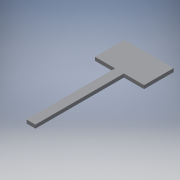
# Autodesk Inventor part: Bevestiging Token
Saved by Autodesk Inventor 2018.3 (Build 223284000, 284)
## iProperties
Created: 2020-12-14
Part Number: Bevestiging Token
Material: Generic
Document SubType Name: Modeling
Designer: daanv
Density: 1 g/cm^3
Appearance: Default
Author: daanv
Autodesk Inventor part; units mm, degrees
ref_plane "YZ Plane" through (0, 0, 0) normal (1, 0, 0) x (0, 1, 0)
ref_plane "XZ Plane" through (0, 0, 0) normal (0, 1, 0) x (-1, 0, 0)
ref_plane "XY Plane" through (0, 0, 0) normal (0, 0, 1) x (1, 0, 0)
sketch "Sketch1" plane through (0, 0, 0) normal (0, 0, 1) x (1, 0, 0)
  line L0 (0, 0) -> (1.8, 0)
  line L1 (1.8, 0) -> (1.8, 18)
  line L2 (1.8, 18) -> (0, 18)
  line L3 (0, 18) -> (0, 0)
  line L4 (-4.1, 18) -> (5.9, 18)
  line L5 (5.9, 18) -> (5.9, 24)
  line L6 (5.9, 24) -> (-4.1, 24)
  line L7 (-4.1, 24) -> (-4.1, 18)
  dimension "d0" = 1.8
  dimension "d1" = 18
  dimension "d2" = 10
  dimension "d3" = 6
  dimension "d4" = 4.1
  dimension "d5" = 4.1
  constraints: 16 end point, 4 parallel, 2 horizontal, 2 perpendicular, 1 point on line
  measures "d0" distance of L2.end L1.end
  measures "d1" distance of L1.end L0.end
  measures "d2" distance of L6.end L5.end
  measures "d3" distance of L5.end L4.end
  measures "d4" distance between parallel lines of L7 L3
  measures "d5" distance between parallel lines of L5 L1
extrude "Extrusion1" add sketch "Sketch1" along normal blind 0.7
body "Solid1"
